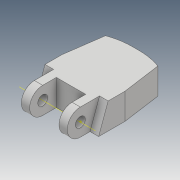
# Autodesk Inventor part: finger_tip
Saved by Autodesk Inventor 2018 (Build 220112000, 112)
## iProperties
Created: 2019-01-30
Part Number: finger_tip
Material: Generic
Document SubType Name: Modeling
Designer: Tsche
Density: 1 g/cm^3
Appearance: Default
Author: Tsche
Autodesk Inventor part; units mm, degrees
ref_plane "YZ Plane" through (0, 0, 0) normal (1, 0, 0) x (0, 1, 0)
ref_plane "XY Plane" through (0, 0, 0) normal (0, 0, 1) x (1, 0, 0)
sketch "Sketch1" plane through (0, 0, 0) normal (0, 0, 1) x (1, 0, 0)
  line L0 (0, -6.0638) -> (7.1374, -6.0638)
  line L1 (7.1374, -6.0638) -> (7.1374, -19.05)
  line L2 (7.1374, -19.05) -> (11.1772, -19.05)
  line L3 (11.1772, -19.05) -> (11.1772, 0)
  line L4 (11.1772, 0) -> (15.367, 0)
  line L5 (15.367, 0) -> (15.367, 4.8514)
  line L6 (15.367, 4.8514) -> (12.7524, 23.4552)
  arc A0 (12.7524, 23.4552) -> (1.5875, 25.4) centre (1.5875, -7.62) ccw
  line L7 (-21.5138, 0) -> (21.5138, 0) construction
  line L8 (0, -28.0365) -> (0, 34.8691) construction
  line L9 (0, -6.0638) -> (-7.1374, -6.0638)
  line L10 (-7.1374, -6.0638) -> (-7.1374, -19.05)
  line L11 (-7.1374, -19.05) -> (-11.1772, -19.05)
  line L12 (-11.1772, -19.05) -> (-11.1772, 0)
  line L13 (-11.1772, 0) -> (-15.367, 0)
  line L14 (-15.367, 0) -> (-15.367, 4.8514)
  line L15 (-15.367, 4.8514) -> (-12.7524, 23.4552)
  line L16 (7.1374, -12.7) -> (11.1772, -12.7) construction
  line L17 (-7.1374, -12.7) -> (-11.1772, -12.7) construction
  line L18 (1.5875, 25.4) -> (0, 25.4)
  arc A1 (-1.5875, 25.4) -> (-12.7524, 23.4552) centre (-1.5875, -7.62) ccw
  line L19 (-1.5875, 25.4) -> (0, 25.4)
  point P0 (0, 0)
  dimension "d1" = 30.734
  dimension "d2" = 4.1898
  dimension "d3" = 4.0398
  dimension "d4" = 6.35
  dimension "d5" = 12.7
  dimension "d6" = 17.5514
  dimension "d7" = 8
  dimension "d8" = 1.5875
  dimension "d9" = 38.1
  dimension "d10" = 33.02
  constraints: 36 end point, 11 horizontal alignment, 6 perpendicular, 4 point on circle, 2 centre point, 2 horizontal, 2 point on line, 1 collinear, 1 equal radius, 1 tangent, 3 other
  measures "d1" distance between parallel lines of L14 L5
  measures "d2" distance of L3.end L4.end
  measures "d3" distance of L1.end L2.end
  measures "d4" distance between parallel lines of L16 L2
  measures "d5" distance between parallel lines of L4 L16
  measures "d6" distance from line of L5.end L16
  measures "d7" angle of L6 L5
  measures "d9" distance between parallel lines of L18 L16
  measures "d10" radius of A0
extrude "Extrusion1" add sketch "Sketch1" along normal blind 12.7
hole "Hole1" at (11.1772, -12.7, 6.35) direction (-1, 0, 0) diameter 4.8006 end through all
fillet "Fillet1" radius 6.35 4 edges at (9.1573, -19.05, 12.7) (9.1573, -19.05, 0) (-9.1573, -19.05, 12.7) (-9.1573, -19.05, 0)
sketch "Sketch2" plane through (11.1772, 0, 12.7) normal (1, 0, 0) x (0, 0, -1)
  line L0 (12.7, 0) -> (0, 0) projected
  line L1 (0, -12.7) -> (0, 0) construction
  line L2 (12.7, -12.7) -> (12.7, 0) construction
  line L3 (0, -3.361) -> (12.7, -7.9834)
  line L4 (12.7, 0) -> (12.7, -7.9834)
  line L5 (0, -3.361) -> (0, 0)
  point P0 (6.35, -12.7)
  dimension "d23" = 6.604
  dimension "d24" = 20
  constraints: 6 end point, 2 collinear, 2 point on line
  measures "d23" distance from line of L3 point (6.35, -12.7)
  measures "d24" angle of L0 L3
extrude "Extrusion2" add sketch "Sketch2" along normal up to surface (4.1898 mm away)
mirror "Mirror1" about plane through (0, 0, 0) normal (1, 0, 0) of "Extrusion2"
ref_plane "Work Plane1" through (0, 0, 6.35) normal (0, 0, -1) x (-1, 0, 0)
ref_plane "Work Plane2" through (11.1772, -12.7, 0) normal (0, 1, 0) x (-1, 0, 0)
equation "\"d1\" = finger_w"
equation "\"d2\" = finger_link_w + tol"
equation "\"d3\" = finger_link_w - tol"
equation "\"d4\" = 0.5 * finger_t"
equation "\"d11\" = finger_t"
equation "\"d15\" = bore_clearance"
equation "\"d22\" = 0.5 * finger_t"
equation "\"d25\" = finger_t"
equation "\"finger_A_l\" = 57.15"
equation "\"finger_w\" = 30.734"
equation "\"finger_B_l\" = 38.1"
equation "\"finger_link_w\" = 4.1148"
equation "\"tolerance1\" = 0.15"
equation "\"tol\" = 0.5 * tolerance1"
equation "\"finger_t\" = 12.7"
equation "\"bore_press\" = 4.8006"
equation "\"bore_clearance\" = bore_press"
body "Solid1"
